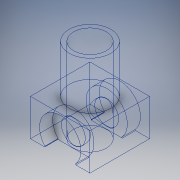
# Autodesk Inventor part: bearingholder
Saved by Autodesk Inventor 2016 (Build 200138000, 138)
## iProperties
Created: 2017-05-27
Part Number: bearingholder
Material: Aluminum 6061
Document SubType Name: Modeling
Designer: Kyle
Mass: 42.5628 g
Surface Area: 97.0119 cm^2
Volume: 15.764 cm^3
Density: 2.7 g/cm^3
Appearance: Aluminum - Flat
Author: Kyle
Autodesk Inventor part; units mm, degrees
ref_plane "YZ Plane" through (0, 0, 0) normal (1, 0, 0) x (0, 1, 0)
ref_plane "XZ Plane" through (0, 0, 0) normal (0, 1, 0) x (-1, 0, 0)
ref_plane "XY Plane" through (0, 0, 0) normal (0, 0, 1) x (1, 0, 0)
sketch "Sketch1" plane through (0, 0, 0) normal (0, 1, 0) x (-1, 0, 0)
  line L0 (0, 0) -> (31.75, 0)
  line L1 (31.75, 0) -> (31.75, -31.75)
  line L2 (31.75, -31.75) -> (0, -31.75)
  line L3 (0, -31.75) -> (0, 0)
  dimension "d0" = 31.75
  dimension "d1" = 31.75
  constraints: 8 end point, 2 parallel, 1 horizontal, 1 perpendicular
  measures "d0" distance of L1.end L2.end
  measures "d1" distance of L0.end L1.end
extrude "Extrusion1" add sketch "Sketch1" along normal blind 19.558
sketch "Sketch2" plane through (0, 19.558, 0) normal (0, 1, 0) x (1, 0, 0)
  line L0 (-31.75, 31.75) -> (-31.75, 0) construction
  line L1 (-31.75, 0) -> (0, 31.75) construction
  circle A0 centre (-15.875, 15.875) radius 11.0808
  point P0 (0, 0)
  dimension "d4" = 22.1615
  constraints: 2 end point, 1 centre point, 1 coincident, 1 midpoint
  measures "d4" diameter of A0
extrude "Extrusion2" add sketch "Sketch2" along normal blind 25.4
sketch "Sketch3" plane through (-15.875, 44.958, -15.875) normal (0, 1, 0) x (1, 0, 0)
  circle A0 centre (0, 0) radius 8.7313
  circle A1 centre (0, 0) radius 11.0808 projected
  point P0 (15.875, -15.875)
  dimension "d19" = 17.4625
  constraints: 1 centre point, 1 coincident
  measures "d19" diameter of A0
extrude "Extrusion3" cut sketch "Sketch3" against normal through all contours A0
sketch "Sketch4" plane through (-31.75, 0, 0) normal (0, 0, 1) x (1, 0, 0)
  circle A0 centre (15.875, 7.796) radius 11
  line L0 (0, 19.558) -> (31.75, 19.558) construction
  line L1 (15.875, 19.558) -> (15.875, 0) construction
  line L2 (31.75, 0) -> (0, 0) construction
  dimension "d10" = 22
  dimension "d20" = 11.762
  constraints: 2 end point, 2 midpoint, 1 centre point, 1 point on line
  measures "d10" diameter of A0
  measures "d20" distance from line of L0 A0.centre
extrude "Extrusion4" cut sketch "Sketch4" against normal blind 7
sketch "Sketch5" plane through (0, 0, -31.75) normal (0, 0, -1) x (-1, 0, 0)
  circle A0 centre (15.875, 7.796) radius 11 projected
  point P0 (0, 0)
extrude "Extrusion5" cut sketch "Sketch5" against normal blind 7
sketch "Sketch6" plane through (-15.875, 7.796, -7) normal (0, 0, 1) x (-1, 0, 0)
  circle A0 centre (0, 0) radius 6.35
  point P0 (-15.875, 7.796)
  dimension "d15" = 12.7
  constraints: 1 centre point
  measures "d15" diameter of A0
extrude "Extrusion6" cut sketch "Sketch6" against normal through all
fillet "Fillet1" radius 0.254 4 edges at (-8.1147, 0, -3.5) (-23.6353, 0, -3.5) (-23.6353, 0, -28.25) (-8.1147, 0, -28.25)
body "Solid1"
